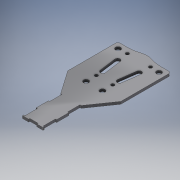
# Autodesk Inventor part: Camera stand plate base
Saved by Autodesk Inventor 2017 (Build 210142000, 142)
## iProperties
Created: 2016-08-03
Part Number: Camera stand plate base
Material: Generic
Document SubType Name: Modeling
Designer: Ali
Density: 1 g/cm^3
Appearance: Default
Author: Ali
Autodesk Inventor part; units mm, degrees
ref_plane "YZ Plane" through (0, 0, 0) normal (1, 0, 0) x (0, 1, 0)
ref_plane "XZ Plane" through (0, 0, 0) normal (0, 1, 0) x (-1, 0, 0)
ref_plane "XY Plane" through (0, 0, 0) normal (0, 0, 1) x (1, 0, 0)
sketch "Sketch1" plane through (0, 0, 0) normal (0, 0, 1) x (1, 0, 0)
  line L0 (-10, -142.3192) -> (-10, -139.3192) projected
  line L1 (-10, -139.3192) -> (10, -139.3192) projected
  line L2 (10, -139.3192) -> (10, -142.3192) projected
  line L3 (10, -142.3192) -> (25, -142.3192) projected
  line L4 (25, -142.3192) -> (25, -139.3192) projected
  line L5 (25, -139.3192) -> (22, -139.3192) projected
  line L6 (22, -139.3192) -> (22, -109.3192) projected
  line L7 (22, -109.3192) -> (25, -109.3192) projected
  line L8 (25, -109.3192) -> (25, -79.3192) projected
  line L9 (25, -79.3192) -> (22, -79.3192) projected
  line L10 (22, -79.3192) -> (22, -49.3192) projected
  line L11 (22, -49.3192) -> (25, -49.3192) projected
  line L12 (25, -49.3192) -> (64.7409, 7.7563) projected
  line L13 (64.7409, 7.7563) -> (64.7409, 124.1392) projected
  arc A0 (64.7409, 124.1392) -> (58.7409, 130.1392) centre (58.7409, 124.1392) ccw projected
  line L14 (58.7409, 130.1392) -> (41.2562, 130.1392) projected
  arc A1 (12.5221, 134.8494) -> (41.2562, 130.1392) centre (41.2562, 220.1392) ccw projected
  arc A2 (12.5221, 134.8494) -> (-12.5221, 134.8494) centre (0, 97.6808) ccw projected
  arc A3 (-41.2562, 130.1392) -> (-12.5221, 134.8494) centre (-41.2562, 220.1392) ccw projected
  line L15 (-41.2562, 130.1392) -> (-58.7409, 130.1392) projected
  arc A4 (-58.7409, 130.1392) -> (-64.7409, 124.1392) centre (-58.7409, 124.1392) ccw projected
  line L16 (-64.7409, 124.1392) -> (-64.7409, 7.7563) projected
  line L17 (-64.7409, 7.7563) -> (-25, -49.3192) projected
  line L18 (-25, -49.3192) -> (-22, -49.3192) projected
  line L19 (-22, -49.3192) -> (-22, -79.3192) projected
  line L20 (-22, -79.3192) -> (-25, -79.3192) projected
  line L21 (-25, -79.3192) -> (-25, -109.3192) projected
  line L22 (-25, -109.3192) -> (-22, -109.3192) projected
  line L23 (-22, -109.3192) -> (-22, -139.3192) projected
  line L24 (-22, -139.3192) -> (-25, -139.3192) projected
  line L25 (-25, -139.3192) -> (-25, -142.3192) projected
  line L26 (-25, -142.3192) -> (-10, -142.3192) projected
  circle A5 centre (-50, 115.7563) radius 3.25 projected
  circle A6 centre (50, 115.7563) radius 3.25 projected
  circle A7 centre (20.018, 7.7563) radius 3.25 projected
  circle A8 centre (-20.018, 7.7563) radius 3.25 projected
  circle A9 centre (-28.3016, 116.7669) radius 4 projected
  circle A10 centre (-20.018, 32.7797) radius 4 projected
  circle A11 centre (20.018, 32.7797) radius 4 projected
  circle A12 centre (28.3016, 116.7669) radius 4 projected
  line L27 (32.1264, 90.1891) -> (26.4217, 48.2224) projected
  arc A13 (14.6157, 49.8272) -> (26.4217, 48.2224) centre (20.5187, 49.0248) ccw projected
  line L28 (14.6157, 49.8272) -> (20.3204, 91.794) projected
  arc A14 (32.1264, 90.1891) -> (20.3204, 91.794) centre (26.2234, 90.9915) ccw projected
  line L29 (-20.3204, 91.794) -> (-14.6157, 49.8272) projected
  arc A15 (-26.4217, 48.2224) -> (-14.6157, 49.8272) centre (-20.5187, 49.0248) ccw projected
  line L30 (-26.4217, 48.2224) -> (-32.1264, 90.1891) projected
  arc A16 (-20.3204, 91.794) -> (-32.1264, 90.1891) centre (-26.2234, 90.9915) ccw projected
  circle A17 centre (50, 115.7563) radius 6.25
  circle A18 centre (-50, 115.7563) radius 6.25
  circle A19 centre (20.018, 7.7563) radius 6.25
  circle A20 centre (-20.018, 7.7563) radius 6.25
  point P0 (0, 0)
  dimension "d0" = 3
  dimension "d1" = 3
  dimension "d2" = 3
  dimension "d3" = 3
  constraints: 4 centre point
  measures "d0" radial gap between concentric circles of A6 A17
  measures "d1" radial gap between concentric circles of A5 A18
  measures "d2" radial gap between concentric circles of A7 A19
  measures "d3" radial gap between concentric circles of A8 A20
extrude "Extrusion1" add sketch "Sketch1" along normal blind 6 contours L26 L25 L24 L23 L22 L21 L20 L19 L18 L17 L16 A4 L15 A3 A2 A1 L14 A0 L13 L12 L11 L10 L9 L8 L7 L6 L5 L4 L3 L2 L1 L0
body "Solid1"
